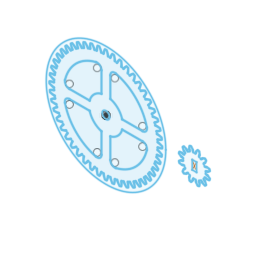
Erasing Gears (Autodesk Fusion 360 design; units mm, degrees)
Autodesk Fusion 360 part; units mm, degrees
(part 1 of 2)
sketch "Sketch1" plane through (0, 0, 0) normal (0, 0, 1) x (1, 0, 0)
  line L0 (60.6226, 5.927) -> (61.428, 6.3048)
  line L1 (59.2748, 5.3967) -> (59.9032, 5.6271)
  line L2 (60.0902, 9.9712) -> (59.3176, 10.0747)
  line L3 (58.5847, -2.5853) -> (58.8217, -2.5026)
  line L4 (62.3136, -6.7626) -> (61.428, -6.2989)
  line L5 (60.1248, 2.2459) -> (59.4717, 2.3923)
  line L6 (63.5931, 1.0414) -> (62.6636, 1.429)
  line L7 (58.8217, 2.5085) -> (58.5847, 2.5911)
  line L8 (62.6636, 1.429) -> (61.725, 1.773)
  line L9 (62.9135, 9.3332) -> (61.9413, 9.5961)
  line L10 (63.1846, -7.2681) -> (62.3136, -6.7626)
  line L11 (59.9032, -5.6212) -> (59.2748, -5.3909)
  line L12 (63.1165, 8.3125) -> (62.9135, 9.3332)
  line L13 (59.4717, -2.3865) -> (60.1248, -2.2401)
  line L14 (59.9032, 5.6271) -> (60.6226, 5.927)
  line L15 (58.5847, 2.5911) -> (58.4674, 2.6941)
  line L16 (58.3185, 4.9664) -> (58.4213, 5.0838)
  line L17 (58.6455, 5.1967) -> (59.2748, 5.3967)
  line L18 (58.4213, 5.0838) -> (58.6455, 5.1967)
  line L19 (59.3176, 10.0747) -> (58.651, 10.1346)
  line L20 (61.428, 6.3048) -> (62.3136, 6.7684)
  line L21 (58.6455, -5.1909) -> (58.4213, -5.078)
  line L22 (62.3136, 6.7684) -> (63.1846, 7.274)
  line L23 (60.9658, 9.8147) -> (60.0902, 9.9712)
  line L24 (59.2748, -5.3909) -> (58.6455, -5.1909)
  line L25 (60.6226, -5.9212) -> (59.9032, -5.6212)
  line L26 (60.8772, -2.0366) -> (61.725, -1.7672)
  line L27 (61.9413, 9.5961) -> (60.9658, 9.8147)
  line L28 (58.3185, -4.9605) -> (58.4674, -2.6883)
  line L29 (63.1846, 7.274) -> (63.1165, 8.3125)
  line L30 (58.4674, -2.6883) -> (58.5847, -2.5853)
  line L31 (58.651, 10.1346) -> (57.9914, 10.1649)
  line L32 (61.725, -1.7672) -> (62.6636, -1.4231)
  line L33 (62.9135, -9.3274) -> (63.1165, -8.3066)
  line L34 (57.0236, 21.4165) -> (57.7037, 21.9898)
  line L35 (58.8217, -2.5026) -> (59.4717, -2.3865)
  line L36 (50.3091, 31.8096) -> (49.6881, 31.5853)
  line L37 (56.3489, 25.2609) -> (55.4626, 25.1854)
  line L38 (58.0636, 13.0876) -> (58.6566, 13.398)
  line L39 (62.6636, -1.4231) -> (63.5931, -1.0356)
  line L40 (52.0297, 27.0555) -> (52.1936, 27.2455)
  line L41 (61.1574, 17.4654) -> (60.1592, 17.5991)
  line L42 (59.1635, 17.6885) -> (58.2749, 17.7294)
  line L43 (56.8268, 17.7043) -> (56.1688, 17.6483)
  line L44 (58.4392, 22.6669) -> (59.1497, 23.3807)
  line L45 (48.6364, 34.3131) -> (49.0654, 34.8268)
  line L46 (53.3852, 24.8293) -> (53.1346, 24.815)
  line L47 (55.3029, 20.1993) -> (55.8589, 20.5554)
  line L48 (52.1936, 27.2455) -> (52.6985, 27.6711)
  line L49 (60.0798, 14.2689) -> (60.8974, 14.8442)
  line L50 (59.1497, 23.3807) -> (58.8152, 24.3661)
  line L51 (61.695, 15.4591) -> (61.4919, 16.4798)
  line L52 (48.1914, 33.8252) -> (48.6364, 34.3131)
  line L53 (49.2885, 31.5689) -> (48.0234, 33.4622)
  line L54 (57.4658, 12.8071) -> (58.0636, 13.0876)
  line L55 (56.1688, 17.6483) -> (55.9185, 17.6668)
  line L56 (48.0234, 33.4622) -> (48.0537, 33.6154)
  line L57 (63.6612, 0.0029) -> (63.5931, 1.0414)
  line L58 (61.428, -6.2989) -> (60.6226, -5.9212)
  line L59 (55.7786, 17.736) -> (55.0466, 19.8922)
  line L60 (60.8772, 2.0425) -> (60.1248, 2.2459)
  line L61 (61.725, 1.773) -> (60.8772, 2.0425)
  line L62 (58.6566, 13.398) -> (59.3307, 13.7892)
  line L63 (54.6896, 25.0854) -> (54.0302, 24.9707)
  line L64 (58.4213, -5.078) -> (58.3185, -4.9605)
  line L65 (58.4674, 2.6941) -> (58.3185, 4.9664)
  line L66 (53.1909, 28.1244) -> (53.7408, 28.6768)
  line L67 (57.9914, 10.1649) -> (57.7456, 10.2159)
  line L68 (56.4063, 20.9406) -> (57.0236, 21.4165)
  line L69 (59.4717, 2.3923) -> (58.8217, 2.5085)
  line L70 (55.0466, 19.8922) -> (55.1155, 20.0323)
  line L71 (52.5701, 32.4) -> (51.7012, 32.2095)
  line L72 (60.8974, 14.8442) -> (61.695, 15.4591)
  line L73 (55.1155, 20.0323) -> (55.3029, 20.1993)
  line L74 (55.5923, 30.9017) -> (55.132, 31.8351)
  line L75 (55.132, 31.8351) -> (54.5538, 32.7005)
  line L76 (53.555, 32.5713) -> (52.5701, 32.4)
  line L77 (60.1248, -2.2401) -> (60.8772, -2.0366)
  line L78 (59.3307, 13.7892) -> (60.0798, 14.2689)
  line L79 (57.7456, 10.2159) -> (57.6159, 10.3027)
  line L80 (57.7037, 21.9898) -> (58.4392, 22.6669)
  line L81 (57.4955, 17.732) -> (56.8268, 17.7043)
  line L82 (55.4626, 25.1854) -> (54.6896, 25.0854)
  line L83 (54.3403, 29.334) -> (54.9811, 30.1013)
  line L84 (57.6159, 10.3027) -> (57.1717, 12.5361)
  line L85 (51.9797, 26.9076) -> (52.0297, 27.0555)
  line L86 (58.8152, 24.3661) -> (58.3548, 25.2996)
  line L87 (57.3477, 25.3022) -> (56.3489, 25.2609)
  line L88 (63.5931, -1.0356) -> (63.6612, 0.0029)
  line L89 (55.9185, 17.6668) -> (55.7786, 17.736)
  line L90 (58.3548, 25.2996) -> (57.3477, 25.3022)
  line L91 (63.1165, -8.3066) -> (63.1846, -7.2681)
  line L92 (52.9868, 24.8653) -> (51.9797, 26.9076)
  line L93 (49.4415, 31.5383) -> (49.2885, 31.5689)
  line L94 (53.7408, 28.6768) -> (54.3403, 29.334)
  line L95 (58.2749, 17.7294) -> (57.4955, 17.732)
  line L96 (48.0537, 33.6154) -> (48.1914, 33.8252)
  line L97 (55.8589, 20.5554) -> (56.4063, 20.9406)
  line L98 (50.5822, 37.0204) -> (51.0837, 37.8938)
  line L99 (32.0044, 50.9529) -> (32.2044, 51.7062)
  line L100 (31.5802, 49.6931) -> (31.8046, 50.3141)
  line L101 (43.7421, 40.368) -> (44.1004, 40.9333)
  line L102 (43.2554, 39.6002) -> (43.3646, 39.8262)
  line L103 (30.8967, 55.5973) -> (30.0963, 54.9861)
  line L104 (40.363, 43.7471) -> (39.8212, 43.3696)
  line L105 (36.1711, 50.052) -> (35.4412, 49.5435)
  line L106 (57.1717, 12.5361) -> (57.2583, 12.666)
  line L107 (44.1004, 40.9333) -> (44.4886, 41.6092)
  line L108 (37.7958, 45.1459) -> (38.0993, 45.7323)
  line L109 (31.8301, 55.137) -> (30.8967, 55.5973)
  line L110 (37.7171, 44.9075) -> (37.7958, 45.1459)
  line L111 (49.5385, 35.4462) -> (50.047, 36.1761)
  line L112 (37.8888, 51.0888) -> (37.0154, 50.5872)
  line L113 (45.3179, 43.3061) -> (45.7012, 44.2375)
  line L114 (38.3808, 46.3395) -> (38.6774, 47.0603)
  line L115 (47.8919, 38.9847) -> (47.0553, 38.6824)
  line L116 (51.7012, 32.2095) -> (50.9479, 32.0095)
  line L117 (44.8975, 42.3992) -> (45.3179, 43.3061)
  line L118 (34.8218, 49.0704) -> (34.3081, 48.6414)
  line L119 (34.3081, 48.6414) -> (33.8202, 48.1964)
  line L120 (61.4919, 16.4798) -> (61.1574, 17.4654)
  line L121 (32.5663, 53.56) -> (32.6954, 54.5588)
  line L122 (51.0837, 37.8938) -> (50.5055, 38.7591)
  line L123 (31.5639, 49.2935) -> (31.5333, 49.4465)
  line L124 (32.2044, 51.7062) -> (32.3949, 52.5751)
  line L125 (50.9479, 32.0095) -> (50.3091, 31.8096)
  line L126 (50.5055, 38.7591) -> (49.8193, 39.5416)
  line L127 (33.4573, 48.0284) -> (31.5639, 49.2935)
  line L128 (43.3011, 45.3229) -> (42.3942, 44.9025)
  line L129 (32.3949, 52.5751) -> (32.5663, 53.56)
  line L130 (54.9811, 30.1013) -> (55.5923, 30.9017)
  line L131 (39.5366, 49.8244) -> (38.7541, 50.5106)
  line L132 (50.047, 36.1761) -> (50.5822, 37.0204)
  line L133 (44.2325, 45.7062) -> (43.3011, 45.3229)
  line L134 (54.5538, 32.7005) -> (53.555, 32.5713)
  line L135 (49.8193, 39.5416) -> (48.8459, 39.2831)
  line L136 (44.4886, 41.6092) -> (44.8975, 42.3992)
  line L137 (54.0302, 24.9707) -> (53.3852, 24.8293)
  line L138 (45.1408, 37.8008) -> (44.9025, 37.722)
  line L139 (44.9025, 37.722) -> (44.7467, 37.7324)
  line L140 (39.5952, 43.2604) -> (39.4394, 43.2504)
  line L141 (38.9797, 47.8969) -> (39.2782, 48.851)
  line L142 (41.6042, 44.4936) -> (40.9283, 44.1054)
  line L143 (31.8046, 50.3141) -> (32.0044, 50.9529)
  line L144 (39.2782, 48.851) -> (39.5366, 49.8244)
  line L145 (44.7467, 37.7324) -> (43.2453, 39.4444)
  line L146 (39.8212, 43.3696) -> (39.5952, 43.2604)
  line L147 (57.2583, 12.666) -> (57.4658, 12.8071)
  line L148 (43.3646, 39.8262) -> (43.7421, 40.368)
  line L149 (60.1592, 17.5991) -> (59.1635, 17.6885)
  line L150 (49.0654, 34.8268) -> (49.5385, 35.4462)
  line L151 (40.9283, 44.1054) -> (40.363, 43.7471)
  line L152 (45.7272, 38.1043) -> (45.1408, 37.8008)
  line L153 (52.6985, 27.6711) -> (53.1909, 28.1244)
  line L154 (42.3942, 44.9025) -> (41.6042, 44.4936)
  line L155 (37.7274, 44.7518) -> (37.7171, 44.9075)
  line L156 (46.3345, 38.3858) -> (45.7272, 38.1043)
  line L157 (53.1346, 24.815) -> (52.9868, 24.8653)
  line L158 (38.0993, 45.7323) -> (38.3808, 46.3395)
  line L159 (39.4394, 43.2504) -> (37.7274, 44.7518)
  line L160 (49.6881, 31.5853) -> (49.4415, 31.5383)
  line L161 (32.6954, 54.5588) -> (31.8301, 55.137)
  line L162 (21.4122, 57.0286) -> (20.9363, 56.4113)
  line L163 (13.7858, 59.3356) -> (13.3946, 58.6615)
  line L164 (25.1805, 55.4676) -> (25.256, 56.3539)
  line L165 (5.0804, 58.4262) -> (4.963, 58.3234)
  line L166 (25.2973, 57.3527) -> (25.2953, 58.3598)
  line L167 (9.9678, 60.0951) -> (9.8113, 60.9708)
  line L168 (25.2953, 58.3598) -> (24.3619, 58.8201)
  line L169 (26.9025, 51.9847) -> (24.8603, 52.9918)
  line L170 (17.7317, 55.7835) -> (17.6625, 55.9235)
  line L171 (27.2405, 52.1986) -> (27.0504, 52.0347)
  line L172 (35.4412, 49.5435) -> (34.8218, 49.0704)
  line L173 (15.4557, 61.6999) -> (14.8408, 60.9023)
  line L174 (12.8037, 57.4707) -> (12.6626, 57.2632)
  line L175 (22.6626, 58.4441) -> (21.9856, 57.7087)
  line L176 (10.0713, 59.3226) -> (9.9678, 60.0951)
  line L177 (8.3091, 63.1215) -> (7.2706, 63.1895)
  line L178 (12.6626, 57.2632) -> (12.5327, 57.1766)
  line L179 (27.0504, 52.0347) -> (26.9025, 51.9847)
  line L180 (10.2993, 57.6208) -> (10.2125, 57.7506)
  line L181 (30.0963, 54.9861) -> (29.329, 54.3453)
  line L182 (5.1933, 58.6504) -> (5.0804, 58.4262)
  line L183 (45.7012, 44.2375) -> (45.0149, 45.02)
  line L184 (38.7541, 50.5106) -> (37.8888, 51.0888)
  line L185 (33.8202, 48.1964) -> (33.6104, 48.0587)
  line L186 (38.6774, 47.0603) -> (38.9797, 47.8969)
  line L187 (27.6661, 52.7035) -> (27.2405, 52.1986)
  line L188 (17.7278, 57.5005) -> (17.726, 58.2799)
  line L189 (12.5327, 57.1766) -> (10.2993, 57.6208)
  line L190 (17.6851, 59.1685) -> (17.5957, 60.1641)
  line L191 (31.5333, 49.4465) -> (31.5802, 49.6931)
  line L192 (45.0149, 45.02) -> (44.2325, 45.7062)
  line L193 (24.81, 53.1396) -> (24.8244, 53.3902)
  line L194 (9.5927, 61.9462) -> (9.3298, 62.9184)
  line L195 (21.9856, 57.7087) -> (21.4122, 57.0286)
  line L196 (47.0553, 38.6824) -> (46.3345, 38.3858)
  line L197 (17.462, 61.1623) -> (16.4764, 61.4969)
  line L198 (5.9236, 60.6275) -> (5.6236, 59.9081)
  line L199 (17.5957, 60.1641) -> (17.462, 61.1623)
  line L200 (48.8459, 39.2831) -> (47.8919, 38.9847)
  line L201 (43.2453, 39.4444) -> (43.2554, 39.6002)
  line L202 (33.6104, 48.0587) -> (33.4573, 48.0284)
  line L203 (13.3946, 58.6615) -> (13.0842, 58.0685)
  line L204 (24.3619, 58.8201) -> (23.3764, 59.1546)
  line L205 (24.8603, 52.9918) -> (24.81, 53.1396)
  line L206 (6.3014, 61.4329) -> (5.9236, 60.6275)
  line L207 (6.765, 62.3185) -> (6.3014, 61.4329)
  line L208 (23.3764, 59.1546) -> (22.6626, 58.4441)
  line L209 (37.0154, 50.5872) -> (36.1711, 50.052)
  line L210 (17.726, 58.2799) -> (17.6851, 59.1685)
  line L211 (10.2125, 57.7506) -> (10.1615, 57.9963)
  line L212 (20.9363, 56.4113) -> (20.5511, 55.8639)
  line L213 (5.6236, 59.9081) -> (5.3933, 59.2797)
  line L214 (9.8113, 60.9708) -> (9.5927, 61.9462)
  line L215 (20.5511, 55.8639) -> (20.1951, 55.3078)
  line L216 (10.1312, 58.6559) -> (10.0713, 59.3226)
  line L217 (29.329, 54.3453) -> (28.6718, 53.7458)
  line L218 (9.3298, 62.9184) -> (8.3091, 63.1215)
  line L219 (20.1951, 55.3078) -> (20.028, 55.1205)
  line L220 (28.6718, 53.7458) -> (28.1194, 53.1959)
  line L221 (10.1615, 57.9963) -> (10.1312, 58.6559)
  line L222 (20.028, 55.1205) -> (19.888, 55.0516)
  line L223 (14.8408, 60.9023) -> (14.2655, 60.0848)
  line L224 (5.3933, 59.2797) -> (5.1933, 58.6504)
  line L225 (24.8244, 53.3902) -> (24.9658, 54.0351)
  line L226 (-20.5521, 55.8626) -> (-20.9373, 56.41)
  line L227 (-5.1942, 58.6491) -> (-5.3942, 59.2784)
  line L228 (-14.2665, 60.0835) -> (-14.8417, 60.901)
  line L229 (25.0805, 54.6946) -> (25.1805, 55.4676)
  line L230 (4.963, 58.3234) -> (2.6907, 58.4723)
  line L231 (-5.9245, 60.6262) -> (-6.3023, 61.4316)
  line L232 (-7.2715, 63.1882) -> (-8.31, 63.1202)
  line L233 (-12.8047, 57.4694) -> (-13.0851, 58.0672)
  line L234 (-2.2435, 60.1284) -> (-2.3899, 59.4753)
  line L235 (-17.6635, 55.9222) -> (-17.7327, 55.7822)
  line L236 (-12.6635, 57.2619) -> (-12.8047, 57.4694)
  line L237 (1.038, 63.5967) -> (-0.0005, 63.6648)
  line L238 (2.5877, 58.5896) -> (2.5051, 58.8266)
  line L239 (-15.4567, 61.6986) -> (-16.4774, 61.4956)
  line L240 (-10.0723, 59.3213) -> (-10.1321, 58.6546)
  line L241 (14.2655, 60.0848) -> (13.7858, 59.3356)
  line L242 (28.1194, 53.1959) -> (27.6661, 52.7035)
  line L243 (-12.5337, 57.1753) -> (-12.6635, 57.2619)
  line L244 (1.7696, 61.7286) -> (1.4256, 62.6672)
  line L245 (-10.3003, 57.6195) -> (-12.5337, 57.1753)
  line L246 (-13.0851, 58.0672) -> (-13.3955, 58.6602)
  line L247 (-14.8417, 60.901) -> (-15.4567, 61.6986)
  line L248 (2.5051, 58.8266) -> (2.3889, 59.4753)
  line L249 (1.4256, 62.6672) -> (1.038, 63.5967)
  line L250 (-5.3942, 59.2784) -> (-5.6246, 59.9068)
  line L251 (-10.2135, 57.7492) -> (-10.3003, 57.6195)
  line L252 (19.888, 55.0516) -> (17.7317, 55.7835)
  line L253 (-6.3023, 61.4316) -> (-6.766, 62.3172)
  line L254 (-9.8123, 60.9695) -> (-9.9688, 60.0938)
  line L255 (-13.7868, 59.3343) -> (-14.2665, 60.0835)
  line L256 (17.7001, 56.8317) -> (17.7278, 57.5005)
  line L257 (-9.5937, 61.9449) -> (-9.8123, 60.9695)
  line L258 (17.6441, 56.1738) -> (17.7001, 56.8317)
  line L259 (16.4764, 61.4969) -> (15.4557, 61.6999)
  line L260 (-2.3899, 59.4753) -> (-2.506, 58.8253)
  line L261 (-1.4265, 62.6672) -> (-1.7706, 61.7286)
  line L262 (-9.9688, 60.0938) -> (-10.0723, 59.3213)
  line L263 (-4.9639, 58.3221) -> (-5.0814, 58.4249)
  line L264 (-16.4774, 61.4956) -> (-17.4629, 61.161)
  line L265 (-21.4132, 57.0273) -> (-21.9865, 57.7074)
  line L266 (-2.506, 58.8253) -> (-2.5887, 58.5883)
  line L267 (-10.1625, 57.995) -> (-10.2135, 57.7492)
  line L268 (-9.3308, 62.9171) -> (-9.5937, 61.9449)
  line L269 (2.2425, 60.1284) -> (2.0391, 60.8808)
  line L270 (25.256, 56.3539) -> (25.2973, 57.3527)
  line L271 (-17.4629, 61.161) -> (-17.5967, 60.1628)
  line L272 (24.9658, 54.0351) -> (25.0805, 54.6946)
  line L273 (-5.6246, 59.9068) -> (-5.9245, 60.6262)
  line L274 (-20.9373, 56.41) -> (-21.4132, 57.0273)
  line L275 (-2.5887, 58.5883) -> (-2.6917, 58.471)
  line L276 (-17.5967, 60.1628) -> (-17.6861, 59.1672)
  line L277 (-5.0814, 58.4249) -> (-5.1942, 58.6491)
  line L278 (-1.7706, 61.7286) -> (-2.04, 60.8808)
  line L279 (2.3889, 59.4753) -> (2.2425, 60.1284)
  line L280 (7.2706, 63.1895) -> (6.765, 62.3185)
  line L281 (13.0842, 58.0685) -> (12.8037, 57.4707)
  line L282 (17.6625, 55.9235) -> (17.6441, 56.1738)
  line L283 (-2.04, 60.8808) -> (-2.2435, 60.1284)
  line L284 (-1.039, 63.5967) -> (-1.4265, 62.6672)
  line L285 (-2.6917, 58.471) -> (-4.9639, 58.3221)
  line L286 (-17.7269, 58.2786) -> (-17.7287, 57.4991)
  line L287 (-17.7287, 57.4991) -> (-17.7011, 56.8304)
  line L288 (2.6907, 58.4723) -> (2.5877, 58.5896)
  line L289 (2.0391, 60.8808) -> (1.7696, 61.7286)
  line L290 (-25.1818, 55.4663) -> (-25.0818, 54.6933)
  line L291 (-24.8113, 53.1383) -> (-24.8616, 52.9905)
  line L292 (-35.4426, 49.5422) -> (-36.1724, 50.0507)
  line L293 (-38.1006, 45.7309) -> (-37.7971, 45.1445)
  line L294 (-31.5652, 49.2921) -> (-33.4586, 48.0271)
  line L295 (-33.4586, 48.0271) -> (-33.6117, 48.0574)
  line L296 (-27.2418, 52.1973) -> (-27.6674, 52.7022)
  line L297 (-17.7011, 56.8304) -> (-17.645, 56.1725)
  line L298 (-6.766, 62.3172) -> (-7.2715, 63.1882)
  line L299 (-26.9039, 51.9834) -> (-27.0518, 52.0334)
  line L300 (-25.2573, 56.3526) -> (-25.1818, 55.4663)
  line L301 (-36.1724, 50.0507) -> (-37.0167, 50.5859)
  line L302 (-0.0005, 63.6648) -> (-1.039, 63.5967)
  line L303 (-20.196, 55.3065) -> (-20.5521, 55.8626)
  line L304 (-37.8901, 51.0875) -> (-38.7554, 50.5093)
  line L305 (-25.0818, 54.6933) -> (-24.9671, 54.0338)
  line L306 (-41.6055, 44.4923) -> (-42.3955, 44.9012)
  line L307 (-38.9811, 47.8956) -> (-38.6787, 47.059)
  line L308 (-13.3955, 58.6602) -> (-13.7868, 59.3343)
  line L309 (-34.8231, 49.0691) -> (-35.4426, 49.5422)
  line L310 (-17.7327, 55.7822) -> (-19.8889, 55.0503)
  line L311 (-10.1321, 58.6546) -> (-10.1625, 57.995)
  line L312 (-44.8988, 42.3979) -> (-44.4899, 41.6079)
  line L313 (-32.5676, 53.5587) -> (-32.3963, 52.5738)
  line L314 (-37.7287, 44.7504) -> (-39.4407, 43.249)
  line L315 (-39.4407, 43.249) -> (-39.5965, 43.2591)
  line L316 (-23.3774, 59.1533) -> (-24.3629, 58.8188)
  line L317 (-33.6117, 48.0574) -> (-33.8215, 48.1951)
  line L318 (-34.3094, 48.6401) -> (-34.8231, 49.0691)
  line L319 (-43.3025, 45.3216) -> (-44.2338, 45.7049)
  line L320 (-37.0167, 50.5859) -> (-37.8901, 51.0875)
  line L321 (-29.3304, 54.344) -> (-30.0976, 54.9848)
  line L322 (-39.2795, 48.8497) -> (-38.9811, 47.8956)
  line L323 (-27.6674, 52.7022) -> (-28.1207, 53.1946)
  line L324 (-30.898, 55.596) -> (-31.8314, 55.1357)
  line L325 (-31.5816, 49.6918) -> (-31.5346, 49.4452)
  line L326 (-32.6968, 54.5575) -> (-32.5676, 53.5587)
  line L327 (-39.8225, 43.3683) -> (-40.3643, 43.7458)
  line L328 (-30.0976, 54.9848) -> (-30.898, 55.596)
  line L329 (-17.645, 56.1725) -> (-17.6635, 55.9222)
  line L330 (-25.2986, 57.3514) -> (-25.2573, 56.3526)
  line L331 (-24.8616, 52.9905) -> (-26.9039, 51.9834)
  line L332 (-24.3629, 58.8188) -> (-25.2963, 58.3585)
  line L333 (-22.6636, 58.4428) -> (-23.3774, 59.1533)
  line L334 (-45.0163, 45.0186) -> (-45.7025, 44.2362)
  line L335 (-17.6861, 59.1672) -> (-17.7269, 58.2786)
  line L336 (-31.8314, 55.1357) -> (-32.6968, 54.5575)
  line L337 (-21.9865, 57.7074) -> (-22.6636, 58.4428)
  line L338 (-27.0518, 52.0334) -> (-27.2418, 52.1973)
  line L339 (-42.3955, 44.9012) -> (-43.3025, 45.3216)
  line L340 (-28.1207, 53.1946) -> (-28.6732, 53.7445)
  line L341 (-20.029, 55.1192) -> (-20.196, 55.3065)
  line L342 (-45.7025, 44.2362) -> (-45.3192, 43.3048)
  line L343 (-28.6732, 53.7445) -> (-29.3304, 54.344)
  line L344 (-24.8257, 53.3889) -> (-24.8113, 53.1383)
  line L345 (-39.5379, 49.8231) -> (-39.2795, 48.8497)
  line L346 (-38.3821, 46.3382) -> (-38.1006, 45.7309)
  line L347 (-25.2963, 58.3585) -> (-25.2986, 57.3514)
  line L348 (-32.3963, 52.5738) -> (-32.2058, 51.7049)
  line L349 (-31.5346, 49.4452) -> (-31.5652, 49.2921)
  line L350 (-8.31, 63.1202) -> (-9.3308, 62.9171)
  line L351 (-32.0058, 50.9516) -> (-31.806, 50.3128)
  line L352 (-39.5965, 43.2591) -> (-39.8225, 43.3683)
  line L353 (-19.8889, 55.0503) -> (-20.029, 55.1192)
  line L354 (-44.7481, 37.7311) -> (-44.9038, 37.7207)
  line L355 (-52.5715, 32.3987) -> (-53.5563, 32.57)
  line L356 (-48.055, 33.6141) -> (-48.0247, 33.4609)
  line L357 (-55.3042, 20.198) -> (-55.1168, 20.031)
  line L358 (-50.3104, 31.8083) -> (-50.9492, 32.0082)
  line L359 (-54.3416, 29.3327) -> (-53.7421, 28.6755)
  line L360 (-24.9671, 54.0338) -> (-24.8257, 53.3889)
  line L361 (-31.806, 50.3128) -> (-31.5816, 49.6918)
  line L362 (-40.3643, 43.7458) -> (-40.9296, 44.1041)
  line L363 (-33.8215, 48.1951) -> (-34.3094, 48.6401)
  line L364 (-32.2058, 51.7049) -> (-32.0058, 50.9516)
  line L365 (-55.8602, 20.5541) -> (-55.3042, 20.198)
  line L366 (-44.9038, 37.7207) -> (-45.1422, 37.7995)
  line L367 (-46.3358, 38.3845) -> (-47.0566, 38.6811)
  line L368 (-52.195, 27.2442) -> (-52.031, 27.0542)
  line L369 (-54.5551, 32.6992) -> (-55.1333, 31.8338)
  line L370 (-49.6894, 31.584) -> (-50.3104, 31.8083)
  line L371 (-52.031, 27.0542) -> (-51.981, 26.9063)
  line L372 (-38.6787, 47.059) -> (-38.3821, 46.3382)
  line L373 (-51.7026, 32.2082) -> (-52.5715, 32.3987)
  line L374 (-57.349, 25.3009) -> (-58.3561, 25.2983)
  line L375 (-56.3502, 25.2596) -> (-57.349, 25.3009)
  line L376 (-43.2568, 39.5989) -> (-43.2467, 39.4431)
  line L377 (-38.7554, 50.5093) -> (-39.5379, 49.8231)
  line L378 (-40.9296, 44.1041) -> (-41.6055, 44.4923)
  line L379 (-53.3865, 24.828) -> (-54.0315, 24.9694)
  line L380 (-45.3192, 43.3048) -> (-44.8988, 42.3979)
  line L381 (-57.705, 21.9885) -> (-57.0249, 21.4152)
  line L382 (-45.7286, 38.103) -> (-46.3358, 38.3845)
  line L383 (-37.7184, 44.9062) -> (-37.7287, 44.7504)
  line L384 (-53.1359, 24.8137) -> (-53.3865, 24.828)
  line L385 (-55.5936, 30.9004) -> (-54.9824, 30.1)
  line L386 (-37.7971, 45.1445) -> (-37.7184, 44.9062)
  line L387 (-48.1927, 33.8239) -> (-48.055, 33.6141)
  line L388 (-58.8164, 24.3649) -> (-59.151, 23.3794)
  line L389 (-48.8473, 39.2818) -> (-49.8207, 39.5403)
  line L390 (-44.2338, 45.7049) -> (-45.0163, 45.0186)
  line L391 (-44.4899, 41.6079) -> (-44.1017, 40.932)
  line L392 (-49.2898, 31.5676) -> (-49.4429, 31.537)
  line L393 (-54.9824, 30.1) -> (-54.3416, 29.3327)
  line L394 (-45.1422, 37.7995) -> (-45.7286, 38.103)
  line L395 (-43.7434, 40.3667) -> (-43.3659, 39.8249)
  line L396 (-55.4639, 25.1841) -> (-56.3502, 25.2596)
  line L397 (-58.4405, 22.6656) -> (-57.705, 21.9885)
  line L398 (-59.3189, 10.0734) -> (-60.0914, 9.9699)
  line L399 (-58.4225, -5.0793) -> (-58.6467, -5.1921)
  line L400 (-49.8207, 39.5403) -> (-50.5069, 38.7578)
  line L401 (-62.6648, -1.4244) -> (-61.7262, -1.7685)
  line L402 (-63.1178, 8.3112) -> (-63.1859, 7.2727)
  line L403 (-50.0484, 36.1748) -> (-49.5398, 35.4449)
  line L404 (-50.9492, 32.0082) -> (-51.7026, 32.2082)
  line L405 (-49.4429, 31.537) -> (-49.6894, 31.584)
  line L406 (-44.1017, 40.932) -> (-43.7434, 40.3667)
  line L407 (-58.0649, 13.0863) -> (-57.4671, 12.8058)
  line L408 (-43.2467, 39.4431) -> (-44.7481, 37.7311)
  line L409 (-53.5563, 32.57) -> (-54.5551, 32.6992)
  line L410 (-57.0249, 21.4152) -> (-56.4076, 20.9393)
  line L411 (-47.8932, 38.9834) -> (-48.8473, 39.2818)
  line L412 (-47.0566, 38.6811) -> (-47.8932, 38.9834)
  line L413 (-48.0247, 33.4609) -> (-49.2898, 31.5676)
  line L414 (-51.981, 26.9063) -> (-52.9881, 24.864)
  line L415 (-43.3659, 39.8249) -> (-43.2568, 39.5989)
  line L416 (-61.4292, 6.3035) -> (-60.6239, 5.9257)
  line L417 (-50.5835, 37.0191) -> (-50.0484, 36.1748)
  line L418 (-58.8229, 2.5072) -> (-59.4729, 2.391)
  line L419 (-63.5944, 1.0401) -> (-63.6624, 0.0016)
  line L420 (-52.9881, 24.864) -> (-53.1359, 24.8137)
  line L421 (-59.276, -5.3921) -> (-59.9044, -5.6225)
  line L422 (-55.1168, 20.031) -> (-55.0479, 19.8909)
  line L423 (-55.0479, 19.8909) -> (-55.7798, 17.7347)
  line L424 (-60.6239, -5.9225) -> (-61.4292, -6.3002)
  line L425 (-62.3148, -6.7639) -> (-63.1859, -7.2694)
  line L426 (-61.6962, 15.4578) -> (-60.8986, 14.8429)
  line L427 (-58.3561, 25.2983) -> (-58.8164, 24.3649)
  line L428 (-55.1333, 31.8338) -> (-55.5936, 30.9004)
  line L429 (-63.5944, -1.0369) -> (-62.6648, -1.4244)
  line L430 (-59.151, 23.3794) -> (-58.4405, 22.6656)
  line L431 (-57.2595, 12.6647) -> (-57.1729, 12.5348)
  line L432 (-60.126, -2.2414) -> (-59.4729, -2.3878)
  line L433 (-53.1923, 28.1231) -> (-52.6998, 27.6698)
  line L434 (-60.8785, 2.0412) -> (-61.7262, 1.7717)
  line L435 (-60.9671, 9.8134) -> (-61.9425, 9.5948)
  line L436 (-48.6377, 34.3118) -> (-48.1927, 33.8239)
  line L437 (-58.3197, -4.9618) -> (-58.4225, -5.0793)
  line L438 (-61.4292, -6.3002) -> (-62.3148, -6.7639)
  line L439 (-49.5398, 35.4449) -> (-49.0668, 34.8255)
  line L440 (-56.828, 17.703) -> (-57.4968, 17.7307)
  line L441 (-53.7421, 28.6755) -> (-53.1923, 28.1231)
  line L442 (-52.6998, 27.6698) -> (-52.195, 27.2442)
  line L443 (-54.6909, 25.0841) -> (-55.4639, 25.1841)
  line L444 (-54.0315, 24.9694) -> (-54.6909, 25.0841)
  line L445 (-56.4076, 20.9393) -> (-55.8602, 20.5541)
  line L446 (-58.5859, 2.5898) -> (-58.8229, 2.5072)
  line L447 (-60.126, 2.2447) -> (-60.8785, 2.0412)
  line L448 (-62.6648, 1.4277) -> (-63.5944, 1.0401)
  line L449 (-57.9926, 10.1636) -> (-58.6523, 10.1333)
  line L450 (-49.0668, 34.8255) -> (-48.6377, 34.3118)
  line L451 (-58.5859, -2.5866) -> (-58.4686, -2.6896)
  line L452 (-63.6624, 0.0016) -> (-63.5944, -1.0369)
  line L453 (-50.5069, 38.7578) -> (-51.0851, 37.8924)
  line L454 (-55.7798, 17.7347) -> (-55.9198, 17.6655)
  line L455 (-60.1605, 17.5978) -> (-61.1587, 17.4641)
  line L456 (-51.0851, 37.8924) -> (-50.5835, 37.0191)
  line L457 (-59.4729, -2.3878) -> (-58.8229, -2.5039)
  line L458 (-59.9044, -5.6225) -> (-60.6239, -5.9225)
  line L459 (-58.3197, 4.9651) -> (-58.4686, 2.6928)
  line L460 (-52.195, -27.2417) -> (-52.6998, -27.6673)
  line L461 (-57.1729, -12.5316) -> (-57.2595, -12.6614)
  line L462 (-57.4968, -17.7278) -> (-56.828, -17.7001)
  line L463 (-60.0811, 14.2676) -> (-59.332, 13.788)
  line L464 (-58.8229, -2.5039) -> (-58.5859, -2.5866)
  line L465 (-57.6172, 10.3014) -> (-57.7469, 10.2146)
  line L466 (-57.7469, 10.2146) -> (-57.9926, 10.1636)
  line L467 (-56.1701, 17.647) -> (-56.828, 17.703)
  line L468 (-61.7262, -1.7685) -> (-60.8785, -2.0379)
  line L469 (-63.1178, -8.3079) -> (-62.9147, -9.3287)
  line L470 (-54.5551, -32.6966) -> (-53.5563, -32.5675)
  line L471 (-60.8785, -2.0379) -> (-60.126, -2.2414)
  line L472 (-53.1359, -24.8111) -> (-52.9881, -24.8614)
  line L473 (-58.6579, 13.3967) -> (-58.0649, 13.0863)
  line L474 (-58.4686, -2.6896) -> (-58.3197, -4.9618)
  line L475 (-59.9044, 5.6258) -> (-59.276, 5.3954)
  line L476 (-60.6239, 5.9257) -> (-59.9044, 5.6258)
  line L477 (-56.4076, -20.9364) -> (-57.0249, -21.4123)
  line L478 (-58.6579, -13.3935) -> (-59.332, -13.7847)
  line L479 (-59.276, 5.3954) -> (-58.6467, 5.1954)
  line L480 (-50.9492, -32.0056) -> (-50.3104, -31.8058)
  line L481 (-57.349, -25.2984) -> (-56.3502, -25.2571)
  line L482 (-58.4405, -22.6627) -> (-59.151, -23.3765)
  line L483 (-58.3561, -25.2954) -> (-57.349, -25.2984)
  line L484 (-60.0811, -14.2644) -> (-60.8986, -14.8396)
  line L485 (-60.9671, -9.8102) -> (-60.0914, -9.9667)
  line L486 (-61.4932, 16.4786) -> (-61.6962, 15.4578)
  line L487 (-52.5715, -32.3961) -> (-51.7026, -32.2056)
  line L488 (-52.9881, -24.8614) -> (-51.981, -26.9037)
  line L489 (-54.6909, -25.0816) -> (-54.0315, -24.9669)
  line L490 (-62.9147, 9.3319) -> (-63.1178, 8.3112)
  line L491 (-51.981, -26.9037) -> (-52.031, -27.0516)
  line L492 (-59.1648, 17.6872) -> (-60.1605, 17.5978)
  line L493 (-61.7262, 1.7717) -> (-62.6648, 1.4277)
  line L494 (-53.5563, -32.5675) -> (-52.5715, -32.3961)
  line L495 (-63.1859, 7.2727) -> (-62.3148, 6.7671)
  line L496 (-58.4225, 5.0825) -> (-58.3197, 4.9651)
  line L497 (-51.7026, -32.2056) -> (-50.9492, -32.0056)
  line L498 (-60.1605, -17.5946) -> (-59.1648, -17.684)
  line L499 (-54.9824, -30.0975) -> (-55.5936, -30.8979)
  line L500 (-55.9198, 17.6655) -> (-56.1701, 17.647)
  line L501 (-54.0315, -24.9669) -> (-53.3865, -24.8254)
  line L502 (-61.6962, -15.4546) -> (-61.4932, -16.4753)
  line L503 (-60.0914, 9.9699) -> (-60.9671, 9.8134)
  line L504 (-58.6523, 10.1333) -> (-59.3189, 10.0734)
  line L505 (-58.6467, 5.1954) -> (-58.4225, 5.0825)
  line L506 (-62.3148, 6.7671) -> (-61.4292, 6.3035)
  line L507 (-59.4729, 2.391) -> (-60.126, 2.2447)
  line L508 (-58.6467, -5.1921) -> (-59.276, -5.3921)
  line L509 (-55.5936, -30.8979) -> (-55.1333, -31.8313)
  line L510 (-55.1333, -31.8313) -> (-54.5551, -32.6966)
  line L511 (-52.031, -27.0516) -> (-52.195, -27.2417)
  line L512 (-61.1587, 17.4641) -> (-61.4932, 16.4786)
  line L513 (-57.9926, -10.1604) -> (-57.7469, -10.2114)
  line L514 (-58.4686, 2.6928) -> (-58.5859, 2.5898)
  line L515 (-59.332, 13.788) -> (-58.6579, 13.3967)
  line L516 (-60.8986, 14.8429) -> (-60.0811, 14.2676)
  line L517 (-61.9425, 9.5948) -> (-62.9147, 9.3319)
  line L518 (-57.4671, 12.8058) -> (-57.2595, 12.6647)
  line L519 (-57.1729, 12.5348) -> (-57.6172, 10.3014)
  line L520 (-58.2762, 17.7281) -> (-59.1648, 17.6872)
  line L521 (-53.3865, -24.8254) -> (-53.1359, -24.8111)
  line L522 (-57.7469, -10.2114) -> (-57.6172, -10.2982)
  line L523 (-57.4968, 17.7307) -> (-58.2762, 17.7281)
  line L524 (-61.4932, -16.4753) -> (-61.1587, -17.4608)
  line L525 (-57.705, -21.9856) -> (-58.4405, -22.6627)
  line L526 (-55.4639, -25.1816) -> (-54.6909, -25.0816)
  line L527 (-49.5398, -35.4424) -> (-50.0484, -36.1723)
  line L528 (-49.8207, -39.5378) -> (-48.8473, -39.2793)
  line L529 (-39.4407, -43.2465) -> (-37.7287, -44.7479)
  line L530 (-37.7287, -44.7479) -> (-37.7184, -44.9037)
  line L531 (-55.0479, -19.8881) -> (-55.1168, -20.0281)
  line L532 (-44.4899, -41.6054) -> (-44.8988, -42.3953)
  line L533 (-48.055, -33.6116) -> (-48.1927, -33.8214)
  line L534 (-39.5965, -43.2566) -> (-39.4407, -43.2465)
  line L535 (-39.2795, -48.8471) -> (-39.5379, -49.8205)
  line L536 (-57.2595, -12.6614) -> (-57.4671, -12.8026)
  line L537 (-59.332, -13.7847) -> (-60.0811, -14.2644)
  line L538 (-57.4671, -12.8026) -> (-58.0649, -13.083)
  line L539 (-34.8231, -49.0666) -> (-34.3094, -48.6376)
  line L540 (-58.0649, -13.083) -> (-58.6579, -13.3935)
  line L541 (-45.7025, -44.2336) -> (-45.0163, -45.0161)
  line L542 (-38.7554, -50.5067) -> (-37.8901, -51.0849)
  line L543 (-48.0247, -33.4584) -> (-48.055, -33.6116)
  line L544 (-45.1422, -37.797) -> (-44.9038, -37.7183)
  line L545 (-49.6894, -31.5814) -> (-49.4429, -31.5345)
  line L546 (-63.1859, -7.2694) -> (-63.1178, -8.3079)
  line L547 (-45.3192, -43.3023) -> (-45.7025, -44.2336)
  line L548 (-57.6172, -10.2982) -> (-57.1729, -12.5316)
  line L549 (-62.9147, -9.3287) -> (-61.9425, -9.5916)
  line L550 (-48.8473, -39.2793) -> (-47.8932, -38.9809)
  line L551 (-34.3094, -48.6376) -> (-33.8215, -48.1926)
  line L552 (-37.0167, -50.5834) -> (-36.1724, -50.0482)
  line L553 (-49.0668, -34.823) -> (-49.5398, -35.4424)
  line L554 (-55.9198, -17.6626) -> (-55.7798, -17.7318)
  line L555 (-55.8602, -20.5512) -> (-56.4076, -20.9364)
  line L556 (-43.3659, -39.8224) -> (-43.7434, -40.3642)
  line L557 (-50.5835, -37.0166) -> (-51.0851, -37.8899)
  line L558 (-59.3189, -10.0702) -> (-58.6523, -10.13)
  line L559 (-53.7421, -28.673) -> (-54.3416, -29.3302)
  line L560 (-58.6523, -10.13) -> (-57.9926, -10.1604)
  line L561 (-55.1168, -20.0281) -> (-55.3042, -20.1952)
  line L562 (-61.9425, -9.5916) -> (-60.9671, -9.8102)
  line L563 (-47.0566, -38.6786) -> (-46.3358, -38.382)
  line L564 (-37.7184, -44.9037) -> (-37.7971, -45.142)
  line L565 (-37.8901, -51.0849) -> (-37.0167, -50.5834)
  line L566 (-60.8986, -14.8396) -> (-61.6962, -15.4546)
  line L567 (-60.0914, -9.9667) -> (-59.3189, -10.0702)
  line L568 (-61.1587, -17.4608) -> (-60.1605, -17.5946)
  line L569 (-56.3502, -25.2571) -> (-55.4639, -25.1816)
  line L570 (-31.5816, -49.6893) -> (-31.806, -50.3103)
  line L571 (-59.1648, -17.684) -> (-58.2762, -17.7248)
  line L572 (-35.4426, -49.5397) -> (-34.8231, -49.0666)
  line L573 (-56.828, -17.7001) -> (-56.1701, -17.6441)
  line L574 (-55.7798, -17.7318) -> (-55.0479, -19.8881)
  line L575 (-46.3358, -38.382) -> (-45.7286, -38.1005)
  line L576 (-58.2762, -17.7248) -> (-57.4968, -17.7278)
  line L577 (-57.0249, -21.4123) -> (-57.705, -21.9856)
  line L578 (-55.3042, -20.1952) -> (-55.8602, -20.5512)
  line L579 (-58.8164, -24.362) -> (-58.3561, -25.2954)
  line L580 (-44.1017, -40.9295) -> (-44.4899, -41.6054)
  line L581 (-51.0851, -37.8899) -> (-50.5069, -38.7553)
  line L582 (-39.8225, -43.3658) -> (-39.5965, -43.2566)
  line L583 (-59.151, -23.3765) -> (-58.8164, -24.362)
  line L584 (-56.1701, -17.6441) -> (-55.9198, -17.6626)
  line L585 (-53.1923, -28.1206) -> (-53.7421, -28.673)
  line L586 (-52.6998, -27.6673) -> (-53.1923, -28.1206)
  line L587 (-54.3416, -29.3302) -> (-54.9824, -30.0975)
  line L588 (-8.31, -63.1177) -> (-7.2715, -63.1858)
  line L589 (-32.5676, -53.5562) -> (-32.6968, -54.555)
  line L590 (-40.3643, -43.7433) -> (-39.8225, -43.3658)
  line L591 (-49.2898, -31.5651) -> (-48.0247, -33.4584)
  line L592 (-43.7434, -40.3642) -> (-44.1017, -40.9295)
  line L593 (-47.8932, -38.9809) -> (-47.0566, -38.6786)
  line L594 (-33.6117, -48.0548) -> (-33.4586, -48.0245)
  line L595 (-33.4586, -48.0245) -> (-31.5652, -49.2896)
  line L596 (-48.6377, -34.3093) -> (-49.0668, -34.823)
  line L597 (-10.1321, -58.6522) -> (-10.0723, -59.3189)
  line L598 (-31.806, -50.3103) -> (-32.0058, -50.9491)
  line L599 (-33.8215, -48.1926) -> (-33.6117, -48.0548)
  line L600 (-45.0163, -45.0161) -> (-44.2338, -45.7023)
  line L601 (-44.8988, -42.3953) -> (-45.3192, -43.3023)
  line L602 (-20.9373, -56.4075) -> (-20.5521, -55.8601)
  line L603 (-50.3104, -31.8058) -> (-49.6894, -31.5814)
  line L604 (-40.9296, -44.1016) -> (-40.3643, -43.7433)
  line L605 (-17.5967, -60.1604) -> (-17.4629, -61.1586)
  line L606 (-10.3003, -57.6171) -> (-10.2135, -57.7468)
  line L607 (-43.2568, -39.5964) -> (-43.3659, -39.8224)
  line L608 (-9.5937, -61.9425) -> (-9.3308, -62.9147)
  line L609 (-38.3821, -46.3357) -> (-38.6787, -47.0565)
  line L610 (-20.029, -55.1167) -> (-19.8889, -55.0478)
  line L611 (-22.6636, -58.4404) -> (-21.9865, -57.7049)
  line L612 (-27.0518, -52.0309) -> (-26.9039, -51.9809)
  line L613 (-24.9671, -54.0314) -> (-25.0818, -54.6908)
  line L614 (-43.2467, -39.4406) -> (-43.2568, -39.5964)
  line L615 (-17.6861, -59.1647) -> (-17.5967, -60.1604)
  line L616 (-23.3774, -59.1509) -> (-22.6636, -58.4404)
  line L617 (-10.2135, -57.7468) -> (-10.1625, -57.9926)
  line L618 (-44.9038, -37.7183) -> (-44.7481, -37.7286)
  line L619 (-32.0058, -50.9491) -> (-32.2058, -51.7024)
  line L620 (-50.0484, -36.1723) -> (-50.5835, -37.0166)
  line L621 (-44.7481, -37.7286) -> (-43.2467, -39.4406)
  line L622 (-25.1818, -55.4638) -> (-25.2573, -56.3501)
  line L623 (-49.4429, -31.5345) -> (-49.2898, -31.5651)
  line L624 (-10.0723, -59.3189) -> (-9.9688, -60.0914)
  line L625 (-25.2573, -56.3501) -> (-25.2986, -57.3489)
  line L626 (-21.9865, -57.7049) -> (-21.4132, -57.0248)
  line L627 (-24.8616, -52.988) -> (-24.8113, -53.1358)
  line L628 (-38.9811, -47.8931) -> (-39.2795, -48.8471)
  line L629 (-31.5346, -49.4427) -> (-31.5816, -49.6893)
  line L630 (-25.2963, -58.356) -> (-24.3629, -58.8164)
  line L631 (-42.3955, -44.8987) -> (-41.6055, -44.4897)
  line L632 (-37.7971, -45.142) -> (-38.1006, -45.7284)
  line L633 (-27.2418, -52.1948) -> (-27.0518, -52.0309)
  line L634 (-41.6055, -44.4897) -> (-40.9296, -44.1016)
  line L635 (-44.2338, -45.7023) -> (-43.3025, -45.3191)
  line L636 (-9.8123, -60.967) -> (-9.5937, -61.9425)
  line L637 (-9.3308, -62.9147) -> (-8.31, -63.1177)
  line L638 (-20.196, -55.3041) -> (-20.029, -55.1167)
  line L639 (-24.8257, -53.3864) -> (-24.9671, -54.0314)
  line L640 (-17.645, -56.17) -> (-17.7011, -56.828)
  line L641 (-43.3025, -45.3191) -> (-42.3955, -44.8987)
  line L642 (-45.7286, -38.1005) -> (-45.1422, -37.797)
  line L643 (-48.1927, -33.8214) -> (-48.6377, -34.3093)
  line L644 (-39.5379, -49.8205) -> (-38.7554, -50.5067)
  line L645 (-38.1006, -45.7284) -> (-38.3821, -46.3357)
  line L646 (-31.5652, -49.2896) -> (-31.5346, -49.4427)
  line L647 (-36.1724, -50.0482) -> (-35.4426, -49.5397)
  line L648 (-38.6787, -47.0565) -> (-38.9811, -47.8931)
  line L649 (-10.1625, -57.9926) -> (-10.1321, -58.6522)
  line L650 (-9.9688, -60.0914) -> (-9.8123, -60.967)
  line L651 (-50.5069, -38.7553) -> (-49.8207, -39.5378)
  line L652 (13.3946, -58.6578) -> (13.7858, -59.3319)
  line L653 (-15.4567, -61.6962) -> (-14.8417, -60.8986)
  line L654 (-19.8889, -55.0478) -> (-17.7327, -55.7798)
  line L655 (-26.9039, -51.9809) -> (-24.8616, -52.988)
  line L656 (5.3933, -59.276) -> (5.6237, -59.9044)
  line L657 (17.6441, -56.17) -> (17.6625, -55.9197)
  line L658 (2.5877, -58.5859) -> (2.6907, -58.4686)
  line L659 (-17.7011, -56.828) -> (-17.7287, -57.4967)
  line L660 (17.462, -61.1586) -> (17.5957, -60.1604)
  line L661 (1.4256, -62.6648) -> (1.7696, -61.7262)
  line L662 (5.6237, -59.9044) -> (5.9236, -60.6238)
  line L663 (7.2706, -63.1858) -> (8.3091, -63.1177)
  line L664 (-12.8047, -57.467) -> (-12.6635, -57.2595)
  line L665 (-31.8314, -55.1332) -> (-30.898, -55.5935)
  line L666 (-5.3942, -59.276) -> (-5.1942, -58.6467)
  line L667 (-25.2986, -57.3489) -> (-25.2963, -58.356)
  line L668 (-20.5521, -55.8601) -> (-20.196, -55.3041)
  line L669 (-2.04, -60.8784) -> (-1.7706, -61.7262)
  line L670 (9.8113, -60.967) -> (9.9678, -60.0914)
  line L671 (2.3889, -59.4729) -> (2.5051, -58.8229)
  line L672 (9.9678, -60.0914) -> (10.0713, -59.3189)
  line L673 (9.5927, -61.9425) -> (9.8113, -60.967)
  line L674 (-28.6732, -53.742) -> (-28.1207, -53.1921)
  line L675 (-1.039, -63.5943) -> (-0.0005, -63.6624)
  line L676 (12.8037, -57.467) -> (13.0842, -58.0648)
  line L677 (-6.3023, -61.4292) -> (-5.9245, -60.6238)
  line L678 (10.1615, -57.9926) -> (10.2125, -57.7468)
  line L679 (-1.4265, -62.6648) -> (-1.039, -63.5943)
  line L680 (14.2655, -60.081) -> (14.8408, -60.8986)
  line L681 (10.2993, -57.6171) -> (12.5327, -57.1729)
  line L682 (-14.8417, -60.8986) -> (-14.2665, -60.081)
  line L683 (17.7278, -57.4967) -> (17.7001, -56.828)
  line L684 (-17.7287, -57.4967) -> (-17.7269, -58.2761)
  line L685 (4.963, -58.3197) -> (5.0804, -58.4225)
  line L686 (-13.7868, -59.3319) -> (-13.3955, -58.6578)
  line L687 (-17.7327, -55.7798) -> (-17.6635, -55.9197)
  line L688 (-17.4629, -61.1586) -> (-16.4774, -61.4931)
  line L689 (13.7858, -59.3319) -> (14.2655, -60.081)
  line L690 (-25.0818, -54.6908) -> (-25.1818, -55.4638)
  line L691 (14.8408, -60.8986) -> (15.4557, -61.6962)
  line L692 (1.7696, -61.7262) -> (2.0391, -60.8784)
  line L693 (2.5051, -58.8229) -> (2.5877, -58.5859)
  line L694 (-32.3963, -52.5713) -> (-32.5676, -53.5562)
  line L695 (-13.3955, -58.6578) -> (-13.0851, -58.0648)
  line L696 (-17.6635, -55.9197) -> (-17.645, -56.17)
  line L697 (-12.6635, -57.2595) -> (-12.5337, -57.1729)
  line L698 (-17.7269, -58.2761) -> (-17.6861, -59.1647)
  line L699 (-27.6674, -52.6997) -> (-27.2418, -52.1948)
  line L700 (-14.2665, -60.081) -> (-13.7868, -59.3319)
  line L701 (-28.1207, -53.1921) -> (-27.6674, -52.6997)
  line L702 (6.3014, -61.4292) -> (6.765, -62.3148)
  line L703 (10.0713, -59.3189) -> (10.1312, -58.6522)
  line L704 (-13.0851, -58.0648) -> (-12.8047, -57.467)
  line L705 (-24.8113, -53.1358) -> (-24.8257, -53.3864)
  line L706 (-30.898, -55.5935) -> (-30.0976, -54.9822)
  line L707 (-21.4132, -57.0248) -> (-20.9373, -56.4075)
  line L708 (-12.5337, -57.1729) -> (-10.3003, -57.6171)
  line L709 (-24.3629, -58.8164) -> (-23.3774, -59.1509)
  line L710 (2.6907, -58.4686) -> (4.963, -58.3197)
  line L711 (-32.2058, -51.7024) -> (-32.3963, -52.5713)
  line L712 (-29.3304, -54.3414) -> (-28.6732, -53.742)
  line L713 (-32.6968, -54.555) -> (-31.8314, -55.1332)
  line L714 (-30.0976, -54.9822) -> (-29.3304, -54.3414)
  line L715 (-16.4774, -61.4931) -> (-15.4567, -61.6962)
  line L716 (27.0504, -52.0309) -> (27.2405, -52.1948)
  line L717 (13.0842, -58.0648) -> (13.3946, -58.6578)
  line L718 (25.1805, -55.4638) -> (25.0805, -54.6908)
  line L719 (20.028, -55.1167) -> (20.1951, -55.3041)
  line L720 (21.9856, -57.7049) -> (22.6626, -58.4404)
  line L721 (26.9026, -51.9809) -> (27.0504, -52.0309)
  line L722 (28.6718, -53.742) -> (29.329, -54.3414)
  line L723 (2.0391, -60.8784) -> (2.2425, -60.126)
  line L724 (-6.766, -62.3148) -> (-6.3023, -61.4292)
  line L725 (33.4573, -48.0245) -> (33.6104, -48.0548)
  line L726 (-7.2715, -63.1858) -> (-6.766, -62.3148)
  line L727 (25.2953, -58.356) -> (25.2973, -57.3489)
  line L728 (6.765, -62.3148) -> (7.2706, -63.1858)
  line L729 (21.4122, -57.0248) -> (21.9856, -57.7049)
  line L730 (25.2973, -57.3489) -> (25.256, -56.3501)
  line L731 (17.7001, -56.828) -> (17.6441, -56.17)
  line L732 (20.5511, -55.8601) -> (20.9363, -56.4075)
  line L733 (-1.7706, -61.7262) -> (-1.4265, -62.6648)
  line L734 (1.038, -63.5943) -> (1.4256, -62.6648)
  line L735 (24.81, -53.1358) -> (24.8603, -52.988)
  line L736 (24.9658, -54.0314) -> (24.8244, -53.3864)
  line L737 (5.9236, -60.6238) -> (6.3014, -61.4292)
  line L738 (16.4765, -61.4931) -> (17.462, -61.1586)
  line L739 (12.6626, -57.2595) -> (12.8037, -57.467)
  line L740 (17.726, -58.2761) -> (17.7278, -57.4967)
  line L741 (-5.6246, -59.9044) -> (-5.3942, -59.276)
  line L742 (-0.0005, -63.6624) -> (1.038, -63.5943)
  line L743 (-2.3899, -59.4729) -> (-2.2435, -60.126)
  line L744 (-2.506, -58.8229) -> (-2.3899, -59.4729)
  line L745 (33.8202, -48.1926) -> (34.3081, -48.6376)
  line L746 (37.0154, -50.5834) -> (37.8888, -51.0849)
  line L747 (39.2782, -48.8471) -> (38.9798, -47.8931)
  line L748 (38.0994, -45.7284) -> (37.7958, -45.142)
  line L749 (17.6851, -59.1647) -> (17.726, -58.2761)
  line L750 (9.3298, -62.9147) -> (9.5927, -61.9425)
  line L751 (38.3808, -46.3357) -> (38.0994, -45.7284)
  line L752 (-5.1942, -58.6467) -> (-5.0814, -58.4225)
  line L753 (37.7958, -45.142) -> (37.7171, -44.9037)
  line L754 (-5.0814, -58.4225) -> (-4.9639, -58.3197)
  line L755 (-2.5887, -58.5859) -> (-2.506, -58.8229)
  line L756 (12.5327, -57.1729) -> (12.6626, -57.2595)
  line L757 (-4.9639, -58.3197) -> (-2.6917, -58.4686)
  line L758 (-5.9245, -60.6238) -> (-5.6246, -59.9044)
  line L759 (-2.6917, -58.4686) -> (-2.5887, -58.5859)
  line L760 (5.1933, -58.6467) -> (5.3933, -59.276)
  line L761 (8.3091, -63.1177) -> (9.3298, -62.9147)
  line L762 (10.2125, -57.7468) -> (10.2993, -57.6171)
  line L763 (-2.2435, -60.126) -> (-2.04, -60.8784)
  line L764 (2.2425, -60.126) -> (2.3889, -59.4729)
  line L765 (37.8888, -51.0849) -> (38.7541, -50.5067)
  line L766 (19.888, -55.0478) -> (20.028, -55.1167)
  line L767 (17.5957, -60.1604) -> (17.6851, -59.1647)
  line L768 (32.6954, -54.555) -> (32.5663, -53.5562)
  line L769 (31.8301, -55.1332) -> (32.6954, -54.555)
  line L770 (23.3764, -59.1509) -> (24.3619, -58.8164)
  line L771 (31.5333, -49.4427) -> (31.5639, -49.2896)
  line L772 (38.7541, -50.5067) -> (39.5366, -49.8205)
  line L773 (5.0804, -58.4225) -> (5.1933, -58.6467)
  line L774 (33.6104, -48.0548) -> (33.8202, -48.1926)
  line L775 (10.1312, -58.6522) -> (10.1615, -57.9926)
  line L776 (15.4557, -61.6962) -> (16.4765, -61.4931)
  line L777 (25.0805, -54.6908) -> (24.9658, -54.0314)
  line L778 (32.5663, -53.5562) -> (32.395, -52.5713)
  line L779 (37.7171, -44.9037) -> (37.7275, -44.7479)
  line L780 (22.6626, -58.4404) -> (23.3764, -59.1509)
  line L781 (53.3853, -24.8254) -> (54.0303, -24.9669)
  line L782 (37.7275, -44.7479) -> (39.4395, -43.2465)
  line L783 (29.329, -54.3414) -> (30.0963, -54.9822)
  line L784 (27.2405, -52.1948) -> (27.6661, -52.6997)
  line L785 (17.7317, -55.7798) -> (19.888, -55.0478)
  line L786 (25.256, -56.3501) -> (25.1805, -55.4638)
  line L787 (54.6897, -25.0816) -> (55.4627, -25.1816)
  line L788 (47.0554, -38.6786) -> (47.892, -38.9809)
  line L789 (43.3012, -45.3191) -> (44.2326, -45.7023)
  line L790 (49.5386, -35.4424) -> (49.0655, -34.823)
  line L791 (44.9026, -37.7183) -> (45.1409, -37.797)
  line L792 (52.5703, -32.3961) -> (53.5551, -32.5675)
  line L793 (58.4393, -22.6627) -> (57.7038, -21.9856)
  line L794 (43.3647, -39.8224) -> (43.2555, -39.5964)
  line L795 (44.7468, -37.7286) -> (44.9026, -37.7183)
  line L796 (53.7409, -28.673) -> (53.191, -28.1206)
  line L797 (39.5953, -43.2566) -> (39.8213, -43.3658)
  line L798 (31.5639, -49.2896) -> (33.4573, -48.0245)
  line L799 (34.3081, -48.6376) -> (34.8218, -49.0666)
  line L800 (34.8218, -49.0666) -> (35.4413, -49.5397)
  line L801 (38.6774, -47.0565) -> (38.3808, -46.3357)
  line L802 (39.8213, -43.3658) -> (40.3631, -43.7433)
  line L803 (20.1951, -55.3041) -> (20.5511, -55.8601)
  line L804 (35.4413, -49.5397) -> (36.1711, -50.0482)
  line L805 (28.1194, -53.1921) -> (28.6718, -53.742)
  line L806 (32.2044, -51.7024) -> (32.0044, -50.9491)
  line L807 (24.8244, -53.3864) -> (24.81, -53.1358)
  line L808 (36.1711, -50.0482) -> (37.0154, -50.5834)
  line L809 (32.0044, -50.9491) -> (31.8046, -50.3103)
  line L810 (50.5823, -37.0166) -> (50.0471, -36.1723)
  line L811 (49.8194, -39.5378) -> (50.5057, -38.7553)
  line L812 (53.5551, -32.5675) -> (54.5539, -32.6966)
  line L813 (57.3479, -25.2984) -> (58.355, -25.2954)
  line L814 (59.1498, -23.3765) -> (58.4393, -22.6627)
  line L815 (45.318, -43.3023) -> (44.8976, -42.3953)
  line L816 (30.8967, -55.5935) -> (31.8301, -55.1332)
  line L817 (39.5366, -49.8205) -> (39.2782, -48.8471)
  line L818 (48.1915, -33.8214) -> (48.0538, -33.6116)
  line L819 (24.3619, -58.8164) -> (25.2953, -58.356)
  line L820 (58.355, -25.2954) -> (58.8153, -24.362)
  line L821 (58.8153, -24.362) -> (59.1498, -23.3765)
  line L822 (54.9812, -30.0975) -> (54.3404, -29.3302)
  line L823 (52.6986, -27.6673) -> (52.1938, -27.2417)
  line L824 (44.1005, -40.9295) -> (43.7422, -40.3642)
  line L825 (32.395, -52.5713) -> (32.2044, -51.7024)
  line L826 (30.0963, -54.9822) -> (30.8967, -55.5935)
  line L827 (46.3346, -38.382) -> (47.0554, -38.6786)
  line L828 (51.0839, -37.8899) -> (50.5823, -37.0166)
  line L829 (48.846, -39.2793) -> (49.8194, -39.5378)
  line L830 (38.9798, -47.8931) -> (38.6774, -47.0565)
  line L831 (31.5802, -49.6893) -> (31.5333, -49.4427)
  line L832 (40.3631, -43.7433) -> (40.9284, -44.1016)
  line L833 (55.4627, -25.1816) -> (56.3491, -25.2571)
  line L834 (49.0655, -34.823) -> (48.6365, -34.3093)
  line L835 (44.2326, -45.7023) -> (45.0151, -45.0161)
  line L836 (27.6661, -52.6997) -> (28.1194, -53.1921)
  line L837 (39.4395, -43.2465) -> (39.5953, -43.2566)
  line L838 (40.9284, -44.1016) -> (41.6043, -44.4897)
  line L839 (24.8603, -52.988) -> (26.9026, -51.9809)
  line L840 (20.9363, -56.4075) -> (21.4122, -57.0248)
  line L841 (17.6625, -55.9197) -> (17.7317, -55.7798)
  line L842 (31.8046, -50.3103) -> (31.5802, -49.6893)
  line L843 (54.0303, -24.9669) -> (54.6897, -25.0816)
  line L844 (61.6951, -15.4546) -> (60.8975, -14.8396)
  line L845 (45.1409, -37.797) -> (45.7273, -38.1005)
  line L846 (52.1938, -27.2417) -> (52.0298, -27.0516)
  line L847 (50.3092, -31.8058) -> (50.948, -32.0056)
  line L848 (50.0471, -36.1723) -> (49.5386, -35.4424)
  line L849 (44.4887, -41.6054) -> (44.1005, -40.9295)
  line L850 (58.6567, -13.3935) -> (58.0637, -13.083)
  line L851 (57.616, -10.2982) -> (57.7457, -10.2114)
  line L852 (59.1637, -17.684) -> (60.1593, -17.5946)
  line L853 (43.2555, -39.5964) -> (43.2454, -39.4406)
  line L854 (51.7014, -32.2056) -> (52.5703, -32.3961)
  line L855 (60.08, -14.2644) -> (59.3308, -13.7847)
  line L856 (55.0467, -19.8881) -> (55.7787, -17.7318)
  line L857 (55.1321, -31.8313) -> (55.5924, -30.8979)
  line L858 (58.2751, -17.7248) -> (59.1637, -17.684)
  line L859 (53.1347, -24.8111) -> (53.3853, -24.8254)
  line L860 (56.8269, -17.7001) -> (57.4956, -17.7278)
  line L861 (56.169, -17.6441) -> (56.8269, -17.7001)
  line L862 (49.6882, -31.5814) -> (50.3092, -31.8058)
  line L863 (44.8976, -42.3953) -> (44.4887, -41.6054)
  line L864 (45.7273, -38.1005) -> (46.3346, -38.382)
  line L865 (56.4065, -20.9364) -> (55.8591, -20.5512)
  line L866 (56.3491, -25.2571) -> (57.3479, -25.2984)
  line L867 (52.0298, -27.0516) -> (51.9798, -26.9037)
  line L868 (47.892, -38.9809) -> (48.846, -39.2793)
  line L869 (58.0637, -13.083) -> (57.4659, -12.8026)
  line L870 (57.0237, -21.4123) -> (56.4065, -20.9364)
  line L871 (57.4956, -17.7278) -> (58.2751, -17.7248)
  line L872 (61.9414, -9.5916) -> (62.9136, -9.3287)
  line L873 (55.1156, -20.0281) -> (55.0467, -19.8881)
  line L874 (43.2454, -39.4406) -> (44.7468, -37.7286)
  line L875 (45.0151, -45.0161) -> (45.7013, -44.2336)
  line L876 (52.987, -24.8614) -> (53.1347, -24.8111)
  line L877 (55.5924, -30.8979) -> (54.9812, -30.0975)
  line L878 (43.7422, -40.3642) -> (43.3647, -39.8224)
  line L879 (53.191, -28.1206) -> (52.6986, -27.6673)
  line L880 (61.4921, -16.4753) -> (61.6951, -15.4546)
  line L881 (50.948, -32.0056) -> (51.7014, -32.2056)
  line L882 (48.0235, -33.4584) -> (49.2886, -31.5651)
  line L883 (45.7013, -44.2336) -> (45.318, -43.3023)
  line L884 (41.6043, -44.4897) -> (42.3943, -44.8987)
  line L885 (42.3943, -44.8987) -> (43.3012, -45.3191)
  line L886 (48.6365, -34.3093) -> (48.1915, -33.8214)
  line L887 (49.2886, -31.5651) -> (49.4416, -31.5345)
  line L888 (50.5057, -38.7553) -> (51.0839, -37.8899)
  line L889 (49.4416, -31.5345) -> (49.6882, -31.5814)
  line L890 (54.5539, -32.6966) -> (55.1321, -31.8313)
  line L891 (54.3404, -29.3302) -> (53.7409, -28.673)
  line L892 (59.3178, -10.0702) -> (60.0903, -9.9667)
  line L893 (51.9798, -26.9037) -> (52.987, -24.8614)
  line L894 (48.0538, -33.6116) -> (48.0235, -33.4584)
  line L895 (61.1575, -17.4608) -> (61.4921, -16.4753)
  line L896 (55.8591, -20.5512) -> (55.303, -20.1952)
  line L897 (57.9915, -10.1604) -> (58.6511, -10.13)
  line L898 (59.3308, -13.7847) -> (58.6567, -13.3935)
  line L899 (60.1593, -17.5946) -> (61.1575, -17.4608)
  line L900 (57.7038, -21.9856) -> (57.0237, -21.4123)
  line L901 (55.303, -20.1952) -> (55.1156, -20.0281)
  line L902 (58.6511, -10.13) -> (59.3178, -10.0702)
  line L903 (57.2584, -12.6614) -> (57.1718, -12.5316)
  line L904 (55.7787, -17.7318) -> (55.9186, -17.6626)
  line L905 (60.0903, -9.9667) -> (60.966, -9.8102)
  line L906 (60.8975, -14.8396) -> (60.08, -14.2644)
  line L907 (62.9136, -9.3287) -> (62.9135, -9.3274)
  line L908 (57.7457, -10.2114) -> (57.9915, -10.1604)
  line L909 (57.4659, -12.8026) -> (57.2584, -12.6614)
  line L910 (57.1718, -12.5316) -> (57.616, -10.2982)
  line L911 (60.966, -9.8102) -> (61.9414, -9.5916)
  line L912 (55.9186, -17.6626) -> (56.169, -17.6441)
  line L913 (98.2624, 14.3913) -> (98.2488, 14.4784)
  line L914 (88.6967, 13.0217) -> (88.0455, 13.1497)
  line L915 (105.8435, 14.9057) -> (105.6254, 16.3014)
  line L916 (105.6907, 13.3328) -> (105.7225, 13.415)
  line L917 (101.7453, 14.132) -> (101.5465, 13.1514)
  line L918 (91.2448, 11.6625) -> (90.8458, 12.0108)
  line L919 (98.0774, 14.9795) -> (97.6083, 15.8299)